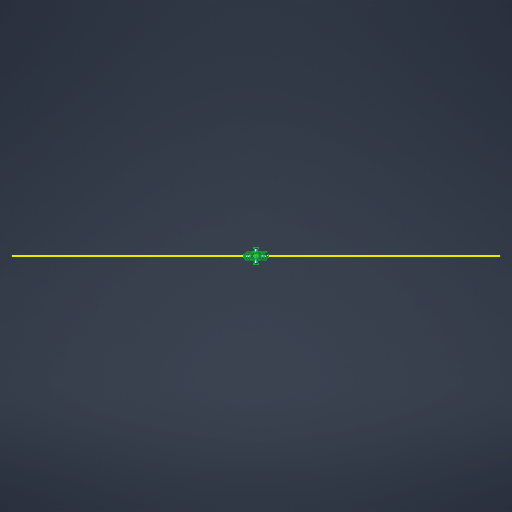
# Autodesk Inventor part: Sensor_Mount
Saved by Autodesk Inventor 2027.1 (Build 311270010, 270A)
## iProperties
Created: 2026-09-08
Part Number: Sensor_Mount
Material: Generic
Document SubType Name: Modeling
Designer: Jacob Parker
Density: 1 g/cm^3
Appearance: Default
Author: Jacob Parker
Autodesk Inventor part; units mm, degrees
ref_plane "YZ Plane" through (0, 0, 0) normal (1, 0, 0) x (0, 1, 0)
ref_plane "XZ Plane" through (0, 0, 0) normal (0, 1, 0) x (-1, 0, 0)
ref_plane "XY Plane" through (0, 0, 0) normal (0, 0, 1) x (1, 0, 0)
sketch "SKbase" plane through (0, 0, 0) normal (0, 1, 0) x (-1, 0, 0)
  line L0 (27.5, 100) -> (-27.5, 100)
  line L1 (-27.5, 100) -> (-27.5, -64)
  line L2 (-27.5, -64) -> (27.5, -64)
  line L3 (27.5, -64) -> (27.5, 100)
  point P0 (0, 0)
  point P1 (27.5, 18)
  dimension "d0" = 55
  dimension "d1" = 164
  constraints: 8 end point, 2 parallel, 1 horizontal, 1 midpoint, 1 other
  measures "d0" distance of L2.end L1.end
  measures "d1" distance of L2.end L0.start
extrude "EXbase" add sketch "SKbase" along normal blind 18
sketch "SKmounting_holes" plane through (0, 0, 0) normal (0, 1, 0) x (1, 0, 0)
  line L0 (0, 147213.6959) -> (0, -147265.0959) projected
  line L1 (-38.5, -19) -> (38.5, -19)
  line L2 (0, -147251.6959) -> (0, 147227.0959)
  line L3 (-27.5, 64) -> (-27.5, -100) projected
  line L4 (-27.5, -100) -> (27.5, -100) projected
  point P0 (0, 0)
  point P1 (-12.5, -94)
  point P2 (-12.5, 56)
  point P3 (12.5, -94)
  point P4 (12.5, 56)
  dimension "d10" = 15
  dimension "d11" = 6
  dimension "d113" = 75
  constraints: 3 vertical alignment, 2 end point, 2 symmetric about line, 3 other
  measures "d10" distance from line of L3 point (-12.5, -94)
  measures "d11" distance from line of L4 point (-12.5, -94)
hole "EXmounting_holes" at (-12.5, 0, 94) at (12.5, 0, 94) at (-12.5, 0, -56) at (12.5, 0, -56) direction (0, 1, 0) diameter 6 end through all
sketch "SKLayout" plane through (0, 18, 0) normal (0, 1, 0) x (1, 0, 0)
  line L0 (-27.5, -86.5) -> (27.5, -86.5)
  line L1 (-27.5, -59.5) -> (27.5, -59.5)
  line L2 (-27.5, 0.5) -> (27.5, 0.5)
  line L3 (-27.5, 64) -> (-27.5, -100) projected
  line L4 (-27.5, 64) -> (27.5, 64)
  line L5 (27.5, -100) -> (27.5, 64) projected
  line L6 (-27.5, -100) -> (27.5, -100) projected
  point P0 (27.5, 64)
  dimension "d81" = 27
  dimension "d82" = 60
  dimension "d109" = 63.5
  dimension "d112" = 13.5
  constraints: 8 end point, 2 point on line, 1 horizontal
  measures "d81" distance between parallel lines of L0 L1
  measures "d82" distance between parallel lines of L1 L2
  measures "d109" distance between parallel lines of L2 L4
  measures "d112" distance between parallel lines of L6 L0
sketch "SKbolt_head_hole" plane through (0, 18, 0) normal (0, 1, 0) x (1, 0, 0)
  point P0 (0, 0)
  point P1 (12.5, 56)
  point P2 (-12.5, 56)
  point P3 (-12.5, -94)
  point P4 (12.5, -94)
hole "Hbolt_head_hole" at (-12.5, 18, 94) at (12.5, 18, 94) at (-12.5, 18, -56) at (12.5, 18, -56) direction (0, -1, 0) diameter 10 depth 5
sketch "SKprint_head_holes" plane through (0, 18, 0) normal (0, 1, 0) x (1, 0, 0)
  circle A0 centre (20, -37) radius 2.5 projected
  circle A1 centre (-20, -53) radius 2.5 projected
  circle A2 centre (-20, -21) radius 2.5 projected
  point P0 (0, 0)
hole "Hprint_head_holes" at (-20, 18, 53) at (-20, 18, 21) at (20, 18, 37) direction (0, -1, 0) diameter 5 end through all
sketch "SKnut_place" plane through (0, 0, 0) normal (0, -1, 0) x (1, 0, 0)
  circle A0 centre (20, 37) radius 2.5 projected
  line L0 (20, 32.75) -> (16.3194, 34.875)
  line L1 (16.3194, 34.875) -> (16.3194, 39.125)
  line L2 (16.3194, 39.125) -> (20, 41.25)
  line L3 (20, 41.25) -> (23.6806, 39.125)
  line L4 (23.6806, 39.125) -> (23.6806, 34.875)
  line L5 (23.6806, 34.875) -> (20, 32.75)
  circle A1 centre (-20, 53) radius 2.5 projected
  line L6 (-20, 48.75) -> (-23.6806, 50.875)
  line L7 (-23.6806, 50.875) -> (-23.6806, 55.125)
  line L8 (-23.6806, 55.125) -> (-20, 57.25)
  line L9 (-20, 57.25) -> (-16.3194, 55.125)
  line L10 (-16.3194, 55.125) -> (-16.3194, 50.875)
  line L11 (-16.3194, 50.875) -> (-20, 48.75)
  circle A2 centre (-20, 21) radius 2.5 projected
  line L12 (-20, 16.75) -> (-23.6806, 18.875)
  line L13 (-23.6806, 18.875) -> (-23.6806, 23.125)
  line L14 (-23.6806, 23.125) -> (-20, 25.25)
  line L15 (-20, 25.25) -> (-16.3194, 23.125)
  line L16 (-16.3194, 23.125) -> (-16.3194, 18.875)
  line L17 (-16.3194, 18.875) -> (-20, 16.75)
  point P0 (0, 0)
  dimension "d97" = 8.5
  dimension "d99" = 8.5
  dimension "d137" = 8.5
  constraints: 36 end point, 3 coincident, 39 other
  measures "d97" distance of L0.start L2.end
  measures "d99" distance of L8.end L6.start
  measures "d137" distance of L14.end L12.start
extrude "EXnut_place" cut sketch "SKnut_place" against normal blind 5.5 contours A0 | L0 L1 L2 L3 L4 L5 | A1 | L6 L7 L8 L9 L10 L11 | A2 | L12 L13 L14 L15 L16 L17
sketch "Sketch13" plane through (0, 0, 0) normal (0, -1, 0) x (1, 0, 0)
  line L0 (-27.5, -0.5) -> (3.5, -0.5) projected
  line L1 (-27.5, -46.5) -> (-27.5, -0.5) projected
  line L2 (3.5, -46.5) -> (-27.5, -46.5) projected
  line L3 (3.5, -0.5) -> (3.5, -46.5) projected
  line L4 (27.5, 100) -> (27.5, -64) projected
  point P0 (0, 0)
  point P1 (27.5, -64)
  point P2 (27.5, -64)
extrude "Extrusion8" cut sketch "Sketch13" against normal blind 12
sketch "Sketch14" plane through (0, 0, 0) normal (0, -1, 0) x (1, 0, 0)
  circle A0 centre (21.5, -93.85) radius 3.25 projected
  circle A1 centre (31.5, -70.15) radius 3.25 projected
  circle A2 centre (11.5, -70.15) radius 3.25 projected
  point P0 (0, 0)
hole "Hole5" at (21.5, 0, -93.85) at (11.5, 0, -70.15) at (31.5, 0, -70.15) direction (0, 1, 0) diameter 6.5 end through all
sketch "Sketch16" plane through (0, 12, 0) normal (0, -1, 0) x (1, 0, 0)
  circle A0 centre (0.4313, -3.5) radius 2 projected
  circle A1 centre (0.4313, -43.5) radius 2 projected
  point P0 (0, 0)
hole "Hole6" at (0.4313, 12, -3.5) at (0.4313, 12, -43.5) direction (0, 1, 0) diameter 4 end through all
fillet "Fillet1" radius 2 4 edges at (0, 18, 100) (-27.5, 18, 18) (27.5, 18, 18) (0, 18, -64)
body "Solid1"
